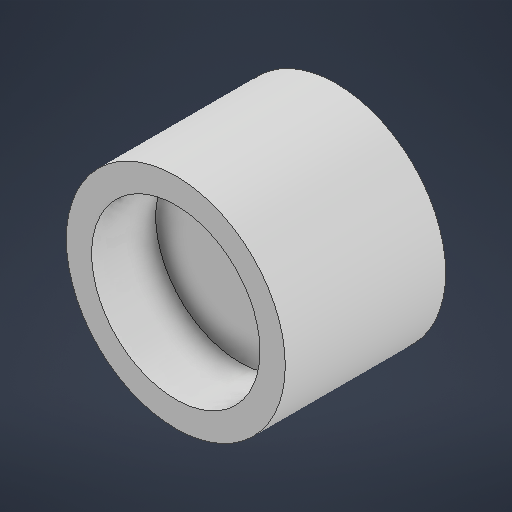
# Autodesk Inventor part: Shaft Coupler
Saved by Autodesk Inventor 2025.3 (Build 293356030, 356C)
## iProperties
Created: 2025-10-14
Part Number: Shaft Coupler
Material: Generic
Document SubType Name: Modeling
Designer: yo
Density: 1 g/cm^3
Appearance: Default
Author: yo
Autodesk Inventor part; units mm, degrees
ref_plane "YZ Plane" through (0, 0, 0) normal (1, 0, 0) x (0, 1, 0)
ref_plane "XZ Plane" through (0, 0, 0) normal (0, 1, 0) x (-1, 0, 0)
ref_plane "XY Plane" through (0, 0, 0) normal (0, 0, 1) x (1, 0, 0)
sketch "Sketch1" plane through (0, 0, 0) normal (0, 0, 1) x (1, 0, 0)
  circle A0 centre (0, 0) radius 5.25
  circle A1 centre (0, 0) radius 6.825
  dimension "d0" = 10.5
  dimension "d1" = 13.65
  constraints: 2 centre point, 2 coincident
  measures "d0" diameter of A0
  measures "d1" diameter of A1
extrude "Extrusion1" add sketch "Sketch1" along normal blind 4
extrude "Extrusion2" add sketch "Sketch1" against normal blind 6 contours A0 | A1
sketch "Sketch2" plane through (0, 0, -6) normal (0, 0, -1) x (-1, 0, 0)
  circle A0 centre (0, 0) radius 3.5
  line L0 (-2.1, 2.8) -> (2.1, 2.8)
  dimension "d6" = 7
  dimension "d7" = 0.7
  constraints: 2 end point, 2 point on circle, 1 centre point, 1 coincident, 1 horizontal
  measures "d6" diameter of A0
  measures "d7" distance edge to line of A0 L0
extrude "Extrusion3" cut sketch "Sketch2" against normal blind 4 contours A0 L0 picked at (-0.6426, 0.8929)
body "Solid1"
